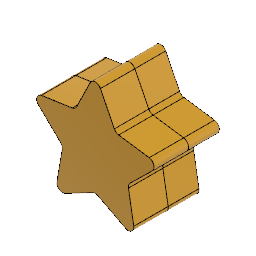
Holly_star v4 (Autodesk Fusion 360 design; units mm, degrees)
Autodesk Fusion 360 part; units mm, degrees
sketch "Sketch1" plane through (0, 0, 0) normal (0, 1, 0) x (1, 0, 0)
  line L0 (0, 0) -> (0, 60) construction
  line L1 (57.0634, 41.459) -> (0, 60) construction
  line L2 (35.2671, 108.541) -> (0, 60) construction
  line L3 (-35.2671, 108.541) -> (0, 60) construction
  line L4 (-57.0634, 41.459) -> (0, 60) construction
  circle A0 centre (-57.0634, 41.459) radius 40 construction
  circle A1 centre (0, 0) radius 40 construction
  line L5 (0, 60) -> (-17.4909, 35.6265) construction
  line L6 (0, 60) -> (17.7756, 35.8333) construction
  line L7 (0, 60) -> (28.4768, 69.4377) construction
  line L8 (0, 60) -> (-0.176, 89.9995) construction
  line L9 (0, 60) -> (-28.5856, 69.103) construction
  line L10 (0, 0) -> (-17.4909, 35.6265)
  line L11 (-17.4909, 35.6265) -> (-57.0634, 41.459)
  line L12 (-28.5856, 69.103) -> (-35.2671, 108.541)
  line L13 (-28.5856, 69.103) -> (-57.0634, 41.459)
  line L14 (-35.2671, 108.541) -> (-0.176, 89.9995)
  line L15 (-0.176, 89.9995) -> (35.2671, 108.541)
  line L16 (35.2671, 108.541) -> (28.4768, 69.4377)
  line L17 (28.4768, 69.4377) -> (57.0634, 41.459)
  line L18 (57.0634, 41.459) -> (17.7756, 35.8333)
  line L19 (17.7756, 35.8333) -> (0, 0)
  dimension "d1" = 60
  dimension "d3" = 360
  dimension "d4" = 80
  dimension "d5" = 80
  dimension "d6" = 30
  dimension "d8" = 360
  constraint coincident L0.start A1.centre
  constraint vertical L0
  constraint coincident L4.start A0.centre
  constraint coincident A0 L5.end
  measures "d1" distance of L0.start L0.end
  measures "d4" diameter of A0
  measures "d5" diameter of A1
  measures "d6" distance of L0.end L5.end
extrude "Extrude1" add sketch "Sketch1" along normal blind 50 makes body 1
fillet "Fillet1" radius 5 10 edges at (57.0634, 25, -41.459) (0, 25, 0) (17.7756, 25, -35.8333) (-57.0634, 25, -41.459) (35.2671, 25, -108.541) (-17.4909, 25, -35.6265) (-28.5856, 25, -69.103) (-35.2671, 25, -108.541) (-0.176, 25, -89.9995) (28.4768, 25, -69.4377) on bodies 1
shell "Shell1" thickness 4 removed faces 1 at (-6.018, 0, -58.0817) on bodies 1
sketch "Sketch2" plane through (0, 0, 0) normal (0, -1, 0) x (1, 0, 0)
  arc A0 (13.0241, -35.2559) -> (19.8109, -40.1656) centre (21.0866, -31.2564) ccw
  line L0 (19.8109, -40.1656) -> (46.4671, -43.9825)
  arc A1 (47.0248, -45.6871) -> (46.4671, -43.9825) centre (46.3254, -44.9724) ccw
  line L1 (47.0248, -45.6871) -> (27.5577, -64.7403)
  arc A2 (27.5577, -64.7403) -> (24.9856, -72.7121) centre (33.8529, -71.1723) ccw
  line L2 (24.9856, -72.7121) -> (29.5927, -99.2432)
  arc A3 (28.1439, -100.3003) -> (29.5927, -99.2432) centre (28.6074, -99.4142) ccw
  line L3 (28.1439, -100.3003) -> (4.0075, -87.6737)
  arc A4 (4.0075, -87.6737) -> (-4.3689, -87.6909) centre (-0.1643, -95.6484) ccw
  line L4 (-4.3689, -87.6909) -> (-28.1778, -100.2711)
  arc A5 (-29.6309, -99.2199) -> (-28.1778, -100.2711) centre (-28.645, -99.387) ccw
  line L5 (-29.6309, -99.2199) -> (-25.0809, -72.363)
  arc A6 (-25.0809, -72.363) -> (-27.6857, -64.4019) centre (-33.9544, -70.8597) ccw
  line L6 (-27.6857, -64.4019) -> (-47.0075, -45.6458)
  arc A7 (-46.4568, -43.9389) -> (-47.0075, -45.6458) centre (-46.311, -44.9282) ccw
  line L7 (-46.4568, -43.9389) -> (-19.5083, -39.967)
  arc A8 (-19.5083, -39.967) -> (-12.7418, -35.0296) centre (-20.8206, -31.0632) ccw
  line L8 (-12.7418, -35.0296) -> (-0.8744, -10.8575)
  arc A9 (0.9191, -10.8538) -> (-0.8744, -10.8575) centre (0.0232, -11.2982) ccw
  line L9 (0.9191, -10.8538) -> (13.0241, -35.2559)
  arc A10 (-33.5747, -98.5518) -> (-26.3091, -103.8078) centre (-28.645, -99.387) ccw
  line L10 (-26.3091, -103.8078) -> (-2.5002, -91.2276)
  arc A11 (2.1533, -91.218) -> (-2.5002, -91.2276) centre (-0.1643, -95.6484) ccw
  line L11 (2.1533, -91.218) -> (26.2897, -103.8446)
  arc A12 (26.2897, -103.8446) -> (33.5337, -98.5588) centre (28.6074, -99.4142) ccw
  line L12 (33.5337, -98.5588) -> (28.9266, -72.0277)
  arc A13 (30.3555, -67.5989) -> (28.9266, -72.0277) centre (33.8529, -71.1723) ccw
  line L13 (30.3555, -67.5989) -> (49.8227, -48.5457)
  arc A14 (49.8227, -48.5457) -> (47.0341, -40.0229) centre (46.3254, -44.9724) ccw
  line L14 (47.0341, -40.0229) -> (20.3778, -36.2059)
  arc A15 (16.6074, -33.4784) -> (20.3778, -36.2059) centre (21.0866, -31.2564) ccw
  line L15 (16.6074, -33.4784) -> (4.5024, -9.0762)
  arc A16 (4.5024, -9.0762) -> (-4.465, -9.0947) centre (0.0232, -11.2982) ccw
  line L16 (-4.465, -9.0947) -> (-16.3324, -33.2668)
  arc A17 (-20.0916, -36.0098) -> (-16.3324, -33.2668) centre (-20.8206, -31.0632) ccw
  line L17 (-20.0916, -36.0098) -> (-47.0401, -39.9817)
  arc A18 (-47.0401, -39.9817) -> (-49.7936, -48.5159) centre (-46.311, -44.9282) ccw
  line L18 (-49.7936, -48.5159) -> (-30.4718, -67.272)
  arc A19 (-29.0247, -71.6949) -> (-30.4718, -67.272) centre (-33.9544, -70.8597) ccw
  line L19 (-29.0247, -71.6949) -> (-33.5747, -98.5518)
  arc A20 (14.8157, -34.3672) -> (20.0944, -38.1858) centre (21.0866, -31.2564) ccw
  line L20 (46.7506, -42.0027) -> (20.0944, -38.1858)
  arc A21 (48.4238, -47.1164) -> (46.7506, -42.0027) centre (46.3254, -44.9724) ccw
  line L21 (28.9566, -66.1696) -> (48.4238, -47.1164)
  arc A22 (28.9566, -66.1696) -> (26.9561, -72.3699) centre (33.8529, -71.1723) ccw
  line L22 (31.5632, -98.901) -> (26.9561, -72.3699)
  arc A23 (27.2168, -102.0725) -> (31.5632, -98.901) centre (28.6074, -99.4142) ccw
  line L23 (3.0804, -89.4459) -> (27.2168, -102.0725)
  arc A24 (3.0804, -89.4459) -> (-3.4346, -89.4593) centre (-0.1643, -95.6484) ccw
  line L24 (-27.2435, -102.0394) -> (-3.4346, -89.4593)
  arc A25 (-31.6028, -98.8858) -> (-27.2435, -102.0394) centre (-28.645, -99.387) ccw
  line L25 (-27.0528, -72.0289) -> (-31.6028, -98.8858)
  arc A26 (-27.0528, -72.0289) -> (-29.0788, -65.8369) centre (-33.9544, -70.8597) ccw
  line L26 (-48.4006, -47.0808) -> (-29.0788, -65.8369)
  arc A27 (-46.7484, -41.9603) -> (-48.4006, -47.0808) centre (-46.311, -44.9282) ccw
  line L27 (-19.8, -37.9884) -> (-46.7484, -41.9603)
  arc A28 (-19.8, -37.9884) -> (-14.5371, -34.1482) centre (-20.8206, -31.0632) ccw
  line L28 (-2.6697, -9.9761) -> (-14.5371, -34.1482)
  arc A29 (2.7107, -9.965) -> (-2.6697, -9.9761) centre (0.0232, -11.2982) ccw
  line L29 (14.8157, -34.3672) -> (2.7107, -9.965)
  dimension "d13" = -2
extrude "Extrude2" cut sketch "Sketch2" against normal blind 23 contours A10 L10 A11 L11 A12 L12 A13 L13 A14 L14 A15 L15 A16 L16 A17 L17 A18 L18 A19 L19 bodies 1
sketch "Sketch3" plane through (0, 23, 0) normal (0, -1, 0) x (1, 0, 0)
  line L0 (48.4238, -47.1164) -> (28.9566, -66.1696)
  arc A0 (28.9566, -66.1696) -> (26.9561, -72.3699) centre (33.8529, -71.1723) ccw
  line L1 (26.9561, -72.3699) -> (31.5632, -98.901)
  arc A1 (27.2168, -102.0725) -> (31.5632, -98.901) centre (28.6074, -99.4142) ccw
  line L2 (27.2168, -102.0725) -> (3.0804, -89.4459)
  arc A2 (3.0804, -89.4459) -> (-3.4346, -89.4593) centre (-0.1643, -95.6484) ccw
  line L3 (-3.4346, -89.4593) -> (-27.2435, -102.0394)
  arc A3 (-31.6028, -98.8858) -> (-27.2435, -102.0394) centre (-28.645, -99.387) ccw
  line L4 (-31.6028, -98.8858) -> (-27.0528, -72.0289)
  arc A4 (-27.0528, -72.0289) -> (-29.0788, -65.8369) centre (-33.9544, -70.8597) ccw
  line L5 (-29.0788, -65.8369) -> (-48.4006, -47.0808)
  arc A5 (-46.7484, -41.9603) -> (-48.4006, -47.0808) centre (-46.311, -44.9282) ccw
  line L6 (-46.7484, -41.9603) -> (-19.8, -37.9884)
  arc A6 (-19.8, -37.9884) -> (-14.5371, -34.1482) centre (-20.8206, -31.0632) ccw
  line L7 (-14.5371, -34.1482) -> (-2.6697, -9.9761)
  arc A7 (2.7107, -9.965) -> (-2.6697, -9.9761) centre (0.0232, -11.2982) ccw
  line L8 (2.7107, -9.965) -> (14.8157, -34.3672)
  arc A8 (14.8157, -34.3672) -> (20.0944, -38.1858) centre (21.0866, -31.2564) ccw
  line L9 (20.0944, -38.1858) -> (46.7506, -42.0027)
  arc A9 (48.4238, -47.1164) -> (46.7506, -42.0027) centre (46.3254, -44.9724) ccw
  line L10 (-20.0916, -36.0098) -> (-47.0401, -39.9817)
  arc A10 (-47.0401, -39.9817) -> (-49.7936, -48.5159) centre (-46.311, -44.9282) ccw
  line L11 (-49.7936, -48.5159) -> (-30.4718, -67.272)
  arc A11 (-29.0247, -71.6949) -> (-30.4718, -67.272) centre (-33.9544, -70.8597) ccw
  line L12 (-29.0247, -71.6949) -> (-33.5747, -98.5518)
  arc A12 (-33.5747, -98.5518) -> (-26.3091, -103.8078) centre (-28.645, -99.387) ccw
  line L13 (-26.3091, -103.8078) -> (-2.5002, -91.2276)
  arc A13 (2.1533, -91.218) -> (-2.5002, -91.2276) centre (-0.1643, -95.6484) ccw
  line L14 (2.1533, -91.218) -> (26.2897, -103.8446)
  arc A14 (26.2897, -103.8446) -> (33.5337, -98.5588) centre (28.6074, -99.4142) ccw
  line L15 (33.5337, -98.5588) -> (28.9266, -72.0277)
  arc A15 (30.3555, -67.5989) -> (28.9266, -72.0277) centre (33.8529, -71.1723) ccw
  line L16 (30.3555, -67.5989) -> (49.8227, -48.5457)
  arc A16 (49.8227, -48.5457) -> (47.0341, -40.0229) centre (46.3254, -44.9724) ccw
  line L17 (47.0341, -40.0229) -> (20.3778, -36.2059)
  arc A17 (16.6074, -33.4784) -> (20.3778, -36.2059) centre (21.0866, -31.2564) ccw
  line L18 (16.6074, -33.4784) -> (4.5024, -9.0762)
  arc A18 (4.5024, -9.0762) -> (-4.465, -9.0947) centre (0.0232, -11.2982) ccw
  line L19 (-4.465, -9.0947) -> (-16.3324, -33.2668)
  arc A19 (-20.0916, -36.0098) -> (-16.3324, -33.2668) centre (-20.8206, -31.0632) ccw
  arc A20 (2.8899, -9.8761) -> (-2.8493, -9.8879) centre (0.0232, -11.2982) ccw
  line L20 (-14.7166, -34.06) -> (-2.8493, -9.8879)
  arc A21 (-19.8291, -37.7906) -> (-14.7166, -34.06) centre (-20.8206, -31.0632) ccw
  line L21 (-46.7776, -41.7624) -> (-19.8291, -37.7906)
  arc A22 (-46.7776, -41.7624) -> (-48.5399, -47.2243) centre (-46.311, -44.9282) ccw
  line L22 (-29.2181, -65.9804) -> (-48.5399, -47.2243)
  arc A23 (-27.25, -71.9955) -> (-29.2181, -65.9804) centre (-33.9544, -70.8597) ccw
  line L23 (-31.8, -98.8524) -> (-27.25, -71.9955)
  arc A24 (-31.8, -98.8524) -> (-27.15, -102.2163) centre (-28.645, -99.387) ccw
  line L24 (-3.3411, -89.6361) -> (-27.15, -102.2163)
  arc A25 (2.9877, -89.6231) -> (-3.3411, -89.6361) centre (-0.1643, -95.6484) ccw
  line L25 (27.1241, -102.2497) -> (2.9877, -89.6231)
  arc A26 (27.1241, -102.2497) -> (31.7602, -98.8668) centre (28.6074, -99.4142) ccw
  line L26 (27.1531, -72.3357) -> (31.7602, -98.8668)
  arc A27 (29.0965, -66.3126) -> (27.1531, -72.3357) centre (33.8529, -71.1723) ccw
  line L27 (48.5637, -47.2593) -> (29.0965, -66.3126)
  arc A28 (48.5637, -47.2593) -> (46.7789, -41.8047) centre (46.3254, -44.9724) ccw
  line L28 (20.1227, -37.9878) -> (46.7789, -41.8047)
  arc A29 (14.9949, -34.2783) -> (20.1227, -37.9878) centre (21.0866, -31.2564) ccw
  line L29 (2.8899, -9.8761) -> (14.9949, -34.2783)
  dimension "d16" = 0.2
extrude "Extrude3" add sketch "Sketch3" along normal blind 24 separate body contours L10 A10 L11 A11 L12 A12 L13 A13 L14 A14 L15 A15 L16 A16 L17 A17 L18 A18 L19 A19 makes body 2
sketch "Sketch4" plane through (0, -1, 0) normal (0, -1, 0) x (1, 0, 0)
  arc A0 (-46.7776, -41.7624) -> (-48.5399, -47.2243) centre (-46.311, -44.9282) ccw
  line L0 (-46.7776, -41.7624) -> (-19.8291, -37.7906)
  arc A1 (-19.8291, -37.7906) -> (-14.7166, -34.06) centre (-20.8206, -31.0632) ccw
  line L1 (-14.7166, -34.06) -> (-2.8493, -9.8879)
  arc A2 (2.8899, -9.8761) -> (-2.8493, -9.8879) centre (0.0232, -11.2982) ccw
  line L2 (2.8899, -9.8761) -> (14.9949, -34.2783)
  arc A3 (14.9949, -34.2783) -> (20.1227, -37.9878) centre (21.0866, -31.2564) ccw
  line L3 (20.1227, -37.9878) -> (46.7789, -41.8047)
  arc A4 (48.5637, -47.2593) -> (46.7789, -41.8047) centre (46.3254, -44.9724) ccw
  line L4 (48.5637, -47.2593) -> (29.0965, -66.3126)
  arc A5 (29.0965, -66.3126) -> (27.1531, -72.3357) centre (33.8529, -71.1723) ccw
  line L5 (27.1531, -72.3357) -> (31.7602, -98.8668)
  arc A6 (27.1241, -102.2497) -> (31.7602, -98.8668) centre (28.6074, -99.4142) ccw
  line L6 (27.1241, -102.2497) -> (2.9877, -89.6231)
  arc A7 (2.9877, -89.6231) -> (-3.3411, -89.6361) centre (-0.1643, -95.6484) ccw
  line L7 (-3.3411, -89.6361) -> (-27.15, -102.2163)
  arc A8 (-31.8, -98.8524) -> (-27.15, -102.2163) centre (-28.645, -99.387) ccw
  line L8 (-31.8, -98.8524) -> (-27.25, -71.9955)
  arc A9 (-27.25, -71.9955) -> (-29.2181, -65.9804) centre (-33.9544, -70.8597) ccw
  line L9 (-29.2181, -65.9804) -> (-48.5399, -47.2243)
  arc A10 (-47.0401, -39.9817) -> (-49.7936, -48.5159) centre (-46.311, -44.9282) ccw
  line L10 (-49.7936, -48.5159) -> (-30.4718, -67.272)
  arc A11 (-29.0247, -71.6949) -> (-30.4718, -67.272) centre (-33.9544, -70.8597) ccw
  line L11 (-29.0247, -71.6949) -> (-33.5747, -98.5518)
  arc A12 (-33.5747, -98.5518) -> (-26.3091, -103.8078) centre (-28.645, -99.387) ccw
  line L12 (-26.3091, -103.8078) -> (-2.5002, -91.2276)
  arc A13 (2.1533, -91.218) -> (-2.5002, -91.2276) centre (-0.1643, -95.6484) ccw
  line L13 (2.1533, -91.218) -> (26.2897, -103.8446)
  arc A14 (26.2897, -103.8446) -> (33.5337, -98.5588) centre (28.6074, -99.4142) ccw
  line L14 (33.5337, -98.5588) -> (28.9266, -72.0277)
  arc A15 (30.3555, -67.5989) -> (28.9266, -72.0277) centre (33.8529, -71.1723) ccw
  line L15 (30.3555, -67.5989) -> (49.8227, -48.5457)
  arc A16 (49.8227, -48.5457) -> (47.0341, -40.0229) centre (46.3254, -44.9724) ccw
  line L16 (47.0341, -40.0229) -> (20.3778, -36.2059)
  arc A17 (16.6074, -33.4784) -> (20.3778, -36.2059) centre (21.0866, -31.2564) ccw
  line L17 (16.6074, -33.4784) -> (4.5024, -9.0762)
  arc A18 (4.5024, -9.0762) -> (-4.465, -9.0947) centre (0.0232, -11.2982) ccw
  line L18 (-4.465, -9.0947) -> (-16.3324, -33.2668)
  arc A19 (-20.0916, -36.0098) -> (-16.3324, -33.2668) centre (-20.8206, -31.0632) ccw
  line L19 (-20.0916, -36.0098) -> (-47.0401, -39.9817)
extrude "Extrude4" add sketch "Sketch4" along normal blind 3 contours A0 L0 A1 L1 A2 L2 A3 L3 A4 L4 A5 L5 A6 L6 A7 L7 A8 L8 A9 L9 | A10 L10 A11 L11 A12 L12 A13 L13 A14 L14 A15 L15 A16 L16 A17 L17 A18 L18 A19 L19 bodies 2
extrude "Extrude5" add 1 faces at (-3.6841, -4, -65.1306) along direction (0, -1, 0) blind 3 on bodies 2 bodies 2
